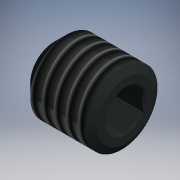
# Autodesk Inventor part: DIN-913 - M3x3
Saved by Autodesk Inventor 2017.3 (Build 213256000, 256)
## iProperties
Part Number: DIN-913 - M3x3
Material: Generic
Catalog Web Link: www.cadenas.de
Description: DIN-913-Gewindestift
Vendor: FESTO
Document SubType Name: Modeling
Designer: partserver
Manufacturer: FESTO
Mass: 0.0175713 g
Surface Area: 0.441289 cm^2
Volume: 0.0175713 cm^3
Density: 1 g/cm^3
Appearance: PSOLRGB-45-51-51
Category: PARTsolutions
Company: FESTO
Title: DIN-913 - M3x3
Author: Cadenas PARTsolutions
Comments: Gewindestift
PSOL_IDENT_0: {$CADENAS_DATA\23d-libs\festo\zyl_zubeh\din_913\din_913.prj},172 {VTYP=3D},{NB=DIN-913 - M3x3},{LINA=
PSOL_IDENT_1: DIN-913 - M3x3},{NN=DIN-913},{DATE=22.07.2016 11:33:17},{GEOMDATE=22.07.2016 11:33:13},{VERSION=v3},
PSOL_IDENT_2: {LINEID=230},{WBVAR=},{WBNUMERIC=}  {NB=DIN-913 - M3x3},{LINA=DIN-913 - M3x3},{KT=X},{IDNR=},{NENN=M
PSOL_IDENT_3: 3x3},{D=3.000},{D3=2.387},{P=0.500},{L=3.000},{DP=2.000},{S=1.500},{T=1.200}
NB: DIN-913 - M3x3
NN: DIN-913
NT: Gewindestift
NBSYN: DIN-913 - $NENN.
LINA: DIN-913 - M3x3
CATALOG: Festo
ROWDESC: M3x3
D: 3
D3: 2.387
P: 0.5
L: 3
DP: 2
S: 1.5
T: 1.2
SUPPLIER: FESTO
ARTICLENO: DIN-913 - M3x3
BOMINFO: DIN-913 - M3x3
CREATOR: CADENAS GmbH
Autodesk Inventor part; units mm, degrees
sketch "Sketch_1" plane through (0, 0, 0) normal (0, 0, 1) x (1, 0, 0)
  line L0 (0.5, 0) -> (3, 0)
  line L1 (3, 0) -> (3, -1)
  line L2 (3, -1) -> (2.5, -1.5)
  line L3 (2.5, -1.5) -> (0.177, -1.5)
  line L4 (0.177, -1.5) -> (0, -1.1935)
  line L5 (0, -1.1935) -> (0, -0.866)
  line L6 (0, -0.866) -> (0.5, 0)
  line L7 (0.5, 0) -> (3, 0)
  constraints: 16 end point
revolve "Revolution1" add sketch "Sketch_1" angle 360 about axis through (0.5, 0, 0) along (1, 0, 0)
thread "Thread1" size "M3x0.5" class "6g" standard "ISO Metric profile" full length
sketch "Sketch_2" plane through (0, 0, 0) normal (1, 0, 0) x (0, 1, 0)
  line L0 (0, 0.866) -> (-0.75, 0.433)
  line L1 (-0.75, 0.433) -> (-0.75, -0.433)
  line L2 (-0.75, -0.433) -> (0, -0.866)
  line L3 (0, -0.866) -> (0.75, -0.433)
  line L4 (0.75, -0.433) -> (0.75, 0.433)
  line L5 (0.75, 0.433) -> (0, 0.866)
  constraints: 12 end point
extrude "Extrusion1" cut sketch "Sketch_2" along normal blind 1.2
ref_plane "IP1_XY" through (0, 0, 0) normal (1, 0, 0) x (0, 0, -1)
ref_plane "IP1_YZ" through (0, 0, 0) normal (0, 0, -1) x (0, 1, 0)
ref_plane "IP1_ZX" through (0, 0, 0) normal (0, 1, 0) x (1, 0, 0)
ref_plane "IP2_XY" through (3, 0, 0) normal (1, 0, 0) x (0, 0, -1)
ref_plane "IP2_YZ" through (3, 0, 0) normal (0, 0, -1) x (0, 1, 0)
ref_plane "IP2_ZX" through (3, 0, 0) normal (0, 1, 0) x (1, 0, 0)
body "Solid1"
